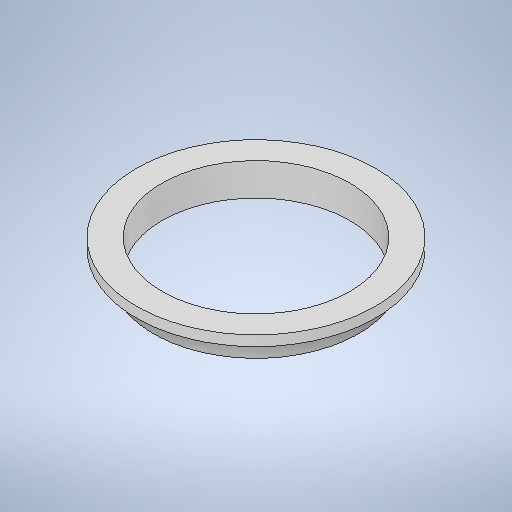
# Autodesk Inventor part: glassSchutz
Saved by Autodesk Inventor 2025.1 (Build 291241000, 241)
## iProperties
Created: 2024-08-07
Part Number: glassSchutz
Material: Generic
Document SubType Name: Modeling
Designer: ffogue
Density: 1 g/cm^3
Appearance: Default
Author: ffogue
Autodesk Inventor part; units mm, degrees
ref_plane "YZ Plane" through (0, 0, 0) normal (1, 0, 0) x (0, 1, 0)
ref_plane "XZ Plane" through (0, 0, 0) normal (0, 1, 0) x (-1, 0, 0)
ref_plane "XY Plane" through (0, 0, 0) normal (0, 0, 1) x (1, 0, 0)
sketch "Sketch1" plane through (0, 0, 0) normal (1, 0, 0) x (0, 0, -1)
  line L0 (-95, 0) -> (-95, 350)
  line L1 (-95, 350) -> (-65, 350)
  line L2 (-65, 350) -> (-65, 300)
  line L3 (-65, 300) -> (0, 300)
  line L4 (0, 300) -> (0, 0)
  line L5 (0, 0) -> (-95, 0)
  dimension "d0" = 700
  dimension "d1" = 600
  dimension "d3" = 65
  dimension "d12" = 30
  constraints: 12 end point, 5 perpendicular, 1 vertical
  measures "d0" diameter of L1 L5
  measures "d1" diameter of L3 L5
  measures "d3" distance of L2.end L3.end
  measures "d12" distance of L0.end L1.end
revolve "Revolution1" add sketch "Sketch1" angle 360 about axis through (0, 0, 0) along (0, 0, 1)
sketch "Sketch2" plane through (0, 0, 0) normal (0, 0, -1) x (-1, 0, 0)
  circle A0 centre (0, 0) radius 300 projected
  point P0 (0, 0)
  constraints: 1 coincident
hole "Hole1" at (0, 0, 0) direction (0, 0, 1) diameter 550 end through all
equation "\"d3\" = glasschudick"
equation "\"glasschudick\" = 65"
body "Solid1"
